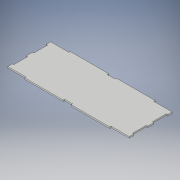
# Autodesk Inventor part: case_roof
Saved by Autodesk Inventor 2019 (Build 230136000, 136)
## iProperties
Created: 2019-07-12
Part Number: case_roof
Material: Generic
Document SubType Name: Modeling
Designer: Lino P
Density: 1 g/cm^3
Appearance: Default
Author: Lino P
Autodesk Inventor part; units mm, degrees
ref_plane "YZ Plane" through (0, 0, 0) normal (1, 0, 0) x (0, 1, 0)
ref_plane "XZ Plane" through (0, 0, 0) normal (0, 1, 0) x (-1, 0, 0)
ref_plane "Work Plane1" through (127, 57.2, 0) normal (0, 1, 0) x (1, 0, 0)
sketch "Sketch3" plane through (127, 57.2, 0) normal (0, 1, 0) x (1, 0, 0)
  line L0 (0, 0) -> (85, 0) construction
  line L1 (0, 0) -> (0, -3) construction
  line L2 (85, -3) -> (0, -3) construction
  line L3 (85, 0) -> (85, -3) construction
  line L4 (-102, 0) -> (-17, 0) construction
  line L5 (-102, 0) -> (-102, -3) construction
  line L6 (-17, -3) -> (-102, -3) construction
  line L7 (-17, 0) -> (-17, -3) construction
  line L8 (122, 10) -> (125, 10) construction
  line L9 (122, 10) -> (122, 0) construction
  line L10 (125, 0) -> (122, 0) construction
  line L11 (125, 10) -> (125, 0) construction
  line L12 (122, 40) -> (125, 40) construction
  line L13 (125, 54) -> (125, 40) construction
  line L14 (122, 54) -> (125, 54) construction
  line L15 (122, 54) -> (122, 40) construction
  line L16 (122, 84) -> (125, 84) construction
  line L17 (125, 94) -> (125, 84) construction
  line L18 (122, 94) -> (125, 94) construction
  line L19 (122, 94) -> (122, 84) construction
  line L20 (122, 0) -> (-139, 0)
  line L21 (-139, 0) -> (-139, 94)
  line L22 (-139, 94) -> (122, 94)
  line L23 (122, 94) -> (122, 0)
  line L24 (-102, 0) -> (-142, 0) projected
  line L25 (-17, -3) -> (-102, -3)
  line L26 (-102, -3) -> (-102, 0)
  line L27 (-102, 0) -> (-17, 0)
  line L28 (-17, 0) -> (-17, -3)
  line L29 (85, -3) -> (0, -3)
  line L30 (0, -3) -> (0, 0)
  line L31 (0, 0) -> (85, 0)
  line L32 (85, 0) -> (85, -3)
  line L33 (122, 10) -> (125, 10) projected
  line L34 (122, 0) -> (125, 0)
  line L35 (125, 0) -> (125, 10)
  line L36 (125, 10) -> (122, 10)
  line L37 (122, 10) -> (122, 0)
  line L38 (125, 54) -> (125, 40) projected
  line L39 (122, 40) -> (125, 40)
  line L40 (125, 40) -> (125, 54)
  line L41 (125, 54) -> (122, 54)
  line L42 (122, 54) -> (122, 40)
  line L43 (122, 94) -> (125, 94)
  line L44 (125, 94) -> (125, 84)
  line L45 (125, 84) -> (122, 84)
  line L46 (122, 84) -> (122, 94)
  line L47 (-139, 47) -> (122, 47) construction
  line L48 (-8.5, 94) -> (-8.5, 0) construction
  line L49 (-139, 10) -> (-142, 10) construction
  line L50 (-139, 10) -> (-139, 0) construction
  line L51 (-142, 0) -> (-139, 0) construction
  line L52 (-142, 10) -> (-142, 0) construction
  line L53 (-139, 40) -> (-142, 40) construction
  line L54 (-142, 54) -> (-142, 40) construction
  line L55 (-139, 54) -> (-142, 54) construction
  line L56 (-139, 54) -> (-139, 40) construction
  line L57 (-139, 84) -> (-142, 84) construction
  line L58 (-142, 94) -> (-142, 84) construction
  line L59 (-139, 94) -> (-142, 94) construction
  line L60 (-139, 94) -> (-139, 84) construction
  line L61 (-139, 94) -> (-139, 0)
  line L62 (-139, 10) -> (-142, 10)
  line L63 (-139, 0) -> (-142, 0)
  line L64 (-142, 0) -> (-142, 10)
  line L65 (-142, 10) -> (-139, 10)
  line L66 (-139, 10) -> (-139, 0)
  line L67 (-142, 54) -> (-142, 40)
  line L68 (-139, 40) -> (-142, 40)
  line L69 (-142, 40) -> (-142, 54)
  line L70 (-142, 54) -> (-139, 54)
  line L71 (-139, 54) -> (-139, 40)
  line L72 (-139, 94) -> (-142, 94)
  line L73 (-142, 94) -> (-142, 84)
  line L74 (-142, 84) -> (-139, 84)
  line L75 (-139, 84) -> (-139, 94)
  line L76 (0, 94) -> (85, 94) construction
  line L77 (0, 94) -> (0, 97) construction
  line L78 (85, 97) -> (0, 97) construction
  line L79 (85, 94) -> (85, 97) construction
  line L80 (-102, 94) -> (-17, 94) construction
  line L81 (-102, 94) -> (-102, 97) construction
  line L82 (-17, 97) -> (-102, 97) construction
  line L83 (-17, 94) -> (-17, 97) construction
  line L84 (-17, 97) -> (-102, 97)
  line L85 (-102, 97) -> (-102, 94)
  line L86 (-102, 94) -> (-17, 94)
  line L87 (-17, 94) -> (-17, 97)
  line L88 (85, 97) -> (0, 97)
  line L89 (0, 97) -> (0, 94)
  line L90 (0, 94) -> (85, 94)
  line L91 (85, 94) -> (85, 97)
  point P0 (-127, 0)
  dimension "d55" = 261
  dimension "d56" = 94
  constraints: 138 end point, 33 symmetric about line, 12 parallel, 6 horizontal, 6 perpendicular, 4 coincident, 4 midpoint
  measures "d55" distance of L21.end L22.end
  measures "d56" distance of L20.end L21.end
extrude "Extrusion4" add sketch "Sketch3" along normal blind 3
body "Solid1"
